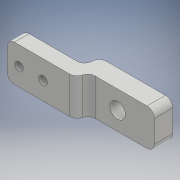
# Autodesk Inventor part: y-endstop-bracket
Saved by Autodesk Inventor 2018 (Build 220112000, 112)
## iProperties
Created: 2018-01-21
Part Number: y-endstop-bracket
Material: Generic
Document SubType Name: Modeling
Designer: Jurjen
Density: 1 g/cm^3
Appearance: Default
Author: Jurjen
Autodesk Inventor part; units mm, degrees
ref_plane "YZ Plane" through (0, 0, 0) normal (1, 0, 0) x (0, 1, 0)
ref_plane "XZ Plane" through (0, 0, 0) normal (0, 1, 0) x (-1, 0, 0)
ref_plane "XY Plane" through (0, 0, 0) normal (0, 0, 1) x (1, 0, 0)
sketch "Sketch1" plane through (0, 0, 0) normal (0, 0, 1) x (1, 0, 0)
  line L0 (-17, 0) -> (0, 0)
  line L1 (-17, -4) -> (-17, 0)
  line L2 (0, 4) -> (20, 4)
  line L3 (20, 4) -> (20, -1)
  line L4 (20, -1) -> (2, -1)
  line L5 (0, 0) -> (0, 4)
  line L6 (0, -4) -> (0, 4) construction
  line L7 (-17, -4) -> (2, -4)
  line L8 (2, -4) -> (2, -1)
  line L9 (0, -4) -> (0, 4) construction
  line L10 (2, -4) -> (2, 4) construction
  point P0 (2, 0)
  dimension "d0" = 5
  dimension "d2" = 4
  dimension "d3" = 20
  dimension "d13" = 19
  dimension "d14" = 2
  dimension "d15" = 4
  constraints: 22 end point, 3 horizontal, 3 midpoint, 3 parallel, 2 perpendicular, 2 vertical, 1 coincident, 1 collinear, 1 horizontal alignment, 1 point on line, 1 vertical alignment
  measures "d0" distance between parallel lines of L4 L2
  measures "d2" distance between parallel lines of L2 L0
  measures "d3" distance between parallel lines of L5 L3
  measures "d13" distance of L1.start L7.end
  measures "d14" distance between parallel lines of L5 L8
  measures "d15" distance between parallel lines of L0 L7
extrude "Extrusion1" add sketch "Sketch1" along normal mid plane 10
sketch "Sketch2" plane through (0, 4, 5) normal (0, 1, 0) x (1, 0, 0)
  circle A0 centre (10, 5) radius 2.1
  line L0 (20, 0) -> (20, 10) projected
  point P0 (0, 5)
  point P1 (20, 5)
  dimension "d7" = 4.2
  dimension "d8" = 10
  constraints: 1 centre point, 1 horizontal alignment, 1 midpoint
  measures "d7" diameter of A0
  measures "d8" distance of A0.centre point (0, 5)
extrude "Extrusion2" cut sketch "Sketch2" against normal through all
fillet "Fillet1" radius 2 4 edges at (0, 0, 0) (0, 4, 0) (2, -4, 0) (2, -1, 0)
sketch "Sketch3" plane through (-17, 0, 5) normal (0, 1, 0) x (1, 0, 0)
  circle A0 centre (9.75, 5.1) radius 1.15
  circle A1 centre (3.25, 5.1) radius 1.15
  line L0 (15, 0) -> (0, 0) projected
  line L1 (0, 10) -> (0, 0) projected
  point P0 (17, 5)
  dimension "d17" = 2.3
  dimension "d18" = 6.5
  dimension "d19" = 5.1
  dimension "d20" = 3.25
  constraints: 2 centre point, 1 equal radius, 1 horizontal alignment
  measures "d17" diameter of A0
  measures "d18" distance of A1.centre A0.centre
  measures "d19" distance from line of A1.centre L0
  measures "d20" distance from line of L1 A1.centre
extrude "Extrusion3" cut sketch "Sketch3" against normal through all
fillet "Fillet2" radius 2 4 edges at (-17, -2, 5) (-17, -2, -5) (20, 1.5, -5) (20, 1.5, 5)
body "Solid1"
